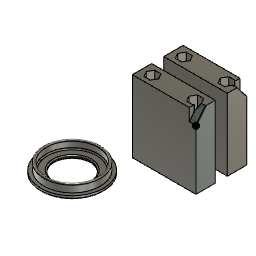
Printer Part v7 (Autodesk Fusion 360 design; units mm, degrees)
Autodesk Fusion 360 part; units mm, degrees
note: some values were not read from the file. Set by a fixed rule: which sketch regions a step uses.
sketch "Sketch1" plane through (0, 0, 0) normal (0, 0, 1) x (1, 0, 0) in component "Left X-Axis Motor Mount"
  line L0 (14.1558, -4.3) -> (-14.1558, -4.3)
  line L1 (-14.1558, -4.3) -> (-14.1558, 4.3)
  line L2 (-14.1558, 4.3) -> (14.1558, 4.3)
  line L3 (14.1558, 4.3) -> (14.1558, -4.3)
  line L4 (14.1558, -4.3) -> (-14.1558, 4.3) construction
  line L5 (-14.1558, -4.3) -> (14.1558, 4.3) construction
  line L6 (-14.1558, 0) -> (14.1558, 0) construction
  circle A0 centre (0, 0) radius 9.5 construction
  line L7 (9.5, 4.3) -> (9.5, -4.3) construction
  line L8 (-9.5, 4.3) -> (-9.5, -4.3) construction
  line L9 (8.1721, 2.3) -> (6.8442, 0)
  line L10 (6.8442, 0) -> (8.1721, -2.3)
  line L11 (8.1721, -2.3) -> (10.8279, -2.3)
  line L12 (10.8279, -2.3) -> (12.1558, 0)
  line L13 (12.1558, 0) -> (10.8279, 2.3)
  line L14 (10.8279, 2.3) -> (8.1721, 2.3)
  line L15 (-10.8279, 2.3) -> (-12.1558, 0)
  line L16 (-12.1558, 0) -> (-10.8279, -2.3)
  line L17 (-10.8279, -2.3) -> (-8.1721, -2.3)
  line L18 (-8.1721, -2.3) -> (-6.8442, 0)
  line L19 (-6.8442, 0) -> (-8.1721, 2.3)
  line L20 (-8.1721, 2.3) -> (-10.8279, 2.3)
  line L21 (8.1144, -2.4) -> (10.8856, -2.4)
  line L22 (10.8856, -2.4) -> (12.2713, 0)
  line L23 (12.2713, 0) -> (10.8856, 2.4)
  line L24 (10.8856, 2.4) -> (8.1144, 2.4)
  line L25 (8.1144, 2.4) -> (6.7287, 0)
  line L26 (6.7287, 0) -> (8.1144, -2.4)
  line L27 (-10.8856, 2.4) -> (-12.2713, 0)
  line L28 (-12.2713, 0) -> (-10.8856, -2.4)
  line L29 (-10.8856, -2.4) -> (-8.1144, -2.4)
  line L30 (-8.1144, -2.4) -> (-6.7287, 0)
  line L31 (-6.7287, 0) -> (-8.1144, 2.4)
  line L32 (-8.1144, 2.4) -> (-10.8856, 2.4)
  point P0 (9.5, 0)
  point P1 (-9.5, 0)
  dimension "d1" = 19
  dimension "d2" = 2.3
  dimension "d3" = 2.3
  dimension "d4" = 2
  dimension "d5" = 2
  dimension "d8" = 0.1
  dimension "d9" = 0.1
  constraint horizontal L0
  constraint perpendicular L0 L1
  constraint parallel L0 L2
  constraint parallel L1 L3
  constraint coincident L4 A0.centre
  constraint coincident L5 A0.centre
  constraint coincident A0.centre origin
  constraint midpoint L1 L6.start
  constraint midpoint L3 L6.end
  constraint coincident L2 L7.start
  constraint coincident L0 L7.end
  constraint perpendicular L0 L7
  constraint coincident L2 L8.start
  constraint coincident L0 L8.end
  constraint perpendicular L0 L8
  constraint tangent A0 L8
  constraint tangent A0 L7
  constraint midpoint L7 P0
  constraint midpoint L8 P1
  constraint perpendicular L7 L14
  constraint perpendicular L8 L20
  measures "d1" diameter of A0
  measures "d2" distance of P0 L14
  measures "d3" distance of P1 L20
  measures "d4" distance of L2 L14
  measures "d5" distance of L3 L12.end
extrude "Extrude1" add sketch "Sketch1" along normal blind 32 contours L0 L1 L2 L3 makes body 1 in component "Left X-Axis Motor Mount"
sketch "Sketch1 (2)" plane through (0, 0, 0) normal (0, 0, 1) x (1, 0, 0) in component "Control Pannel Knob Light Sheld"
  circle A0 centre (0, 0) radius 14
  circle A1 centre (0, 0) radius 8
  dimension "d10" = 28
  dimension "d11" = 16
  constraint coincident A0.centre A1.centre
  measures "d10" diameter of A0
  measures "d11" diameter of A1
extrude "Extrude1'" add sketch "Sketch1 (2)" along normal blind 1.5 separate body makes body 2 in component "Control Pannel Knob Light Sheld"
sketch "Sketch2" plane through (0, 0, 1.5) normal (0, 0, 1) x (-1, 0, 0) in component "Control Pannel Knob Light Sheld"
  circle A0 centre (0, 0) radius 8
  circle A1 centre (0, 0) radius 14
  circle A2 centre (0, 0) radius 12.5
  circle A3 centre (0, 0) radius 11.5
  dimension "d14" = 25
  dimension "d15" = 23
  constraint coincident A0.centre A1.centre
  constraint concentric A2 A3
  measures "d14" diameter of A2
  measures "d15" diameter of A3
extrude "Extrude2" add sketch "Sketch2" along normal blind 3.5 contours A2 bodies 2 in component "Control Pannel Knob Light Sheld"
fillet "Fillet1" radius 0.5 6 edges at (-13.0526, -5.0626, 0) (-7.4586, 2.8929, 0) (-7.4586, 2.8929, 1.5) (11.6541, 4.5202, 5) (10.7218, -4.1586, 5) (10.7218, 4.1586, 1.5) on bodies 2 in component "Control Pannel Knob Light Sheld"
sketch "Sketch2 (2)" plane through (14.1558, 0, 0) normal (1, 0, 0) x (0, 1, 0) in component "Left X-Axis Motor Mount"
  line L0 (-4.3, 0) -> (4.3, 0)
  line L1 (4.3, 0) -> (4.3, 32)
  line L2 (4.3, 32) -> (-4.3, 32)
  line L3 (-4.3, 32) -> (-4.3, 0)
  line L4 (0, 32) -> (-4.3, 26.4764)
  dimension "d23" = 7
  constraint midpoint L2 L4.start
  constraint coincident L3 L4.end
  measures "d23" distance of L4.start L4.end
copy_body "CopyPasteBodies1" bodies 1 body 1 seen with x (1, 0, 0) y (0, 1, 0) z (0, 0, 1) at (23.5407, 21.7309, 2.2514) makes body 3 in component "Right X-Axis Motor Mount"
move_body "Move1" bodies 3 to x (1, 0, 0) y (0, 1, 0) z (0, 0, 1) at (0, 14, 0) in component "Right X-Axis Motor Mount"
sketch "Sketch1 (3)" plane through (37.6965, 0, 0) normal (1, 0, 0) x (0, 1, 0) in component "Right X-Axis Motor Mount"
  line L0 (31.4309, 2.2514) -> (40.0309, 2.2514)
  line L1 (40.0309, 2.2514) -> (40.0309, 34.2514)
  line L2 (40.0309, 34.2514) -> (31.4309, 34.2514)
  line L3 (31.4309, 34.2514) -> (31.4309, 2.2514)
  line L4 (35.7309, 34.2514) -> (40.0309, 28.7278)
  dimension "d22" = 7
  constraint midpoint L2 L4.start
  constraint coincident L1 L4.end
  measures "d22" distance of L4.start L4.end
extrude "Extrude3" cut sketch "Sketch2 (2)" against normal blind 3 contours L2 L3 L4 bodies 1 in component "Left X-Axis Motor Mount"
extrude "Extrude1''" cut sketch "Sketch1 (3)" against normal blind 3 contours L1 L2 L4 bodies 3 in component "Right X-Axis Motor Mount"
extrude "Extrude2'" cut sketch "Sketch2 (2)" against normal blind 3 contours L2 L3 L4 bodies 1 in component "Left X-Axis Motor Mount"
component "Left X-Axis Motor Mount" placed x (1, 0, 0) y (0, 1, 0) z (0, 0, 1) at (23.5407, 21.7309, 2.2514)
component "Control Pannel Knob Light Sheld" placed x (1, 0, 0) y (0, 1, 0) z (0, 0, 1) at (0, 0, 0)
component "Right X-Axis Motor Mount" placed x (1, 0, 0) y (0, 1, 0) z (0, 0, 1) at (0, 0, 0)
equation "d2 = ( 4.6 / 2 ) * 1 mm"
equation "d3 = ( 4.6 / 2 ) * 1 mm"
